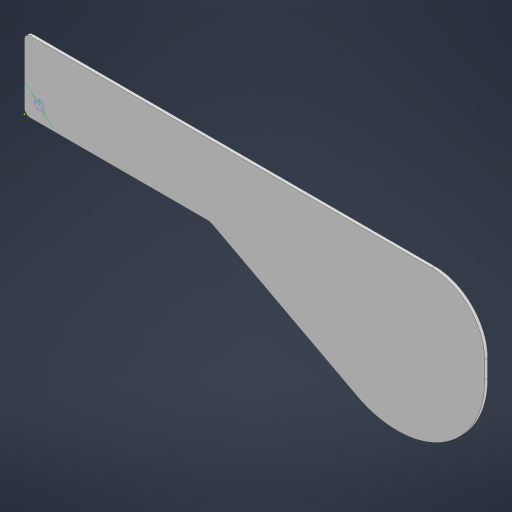
# Autodesk Inventor part: intake sled v5
Saved by Autodesk Inventor 2023.4 (Build 274418000, 418)
## iProperties
Created: 2023-12-16
Part Number: intake sled v5
Material: Generic
Document SubType Name: Modeling
Designer: Meer
Density: 1 g/cm^3
Appearance: Default
Author: Meer
Autodesk Inventor part; units mm, degrees
ref_plane "YZ Plane" through (0, 0, 0) normal (1, 0, 0) x (0, 1, 0)
ref_plane "XZ Plane" through (0, 0, 0) normal (0, 1, 0) x (-1, 0, 0)
ref_plane "XY Plane" through (0, 0, 0) normal (0, 0, 1) x (1, 0, 0)
sketch "Sketch1" plane through (0, 0, 0) normal (0, 0, 1) x (1, 0, 0)
  line L0 (0, 0) -> (247.65, 0)
  line L1 (247.65, 0) -> (247.65, 38.1)
  line L2 (247.65, 38.1) -> (0, 38.1)
  line L3 (0, 38.1) -> (0, 0)
  line L4 (286.1616, 0) -> (255.1962, 0)
  line L5 (255.1962, 0) -> (255.1962, 12.7)
  line L6 (255.1962, 12.7) -> (286.1616, 12.7)
  line L7 (286.1616, 12.7) -> (286.1616, 0)
  line L8 (247.65, 12.7) -> (200.66, 12.7)
  circle A0 centre (200.6294, 0) radius 47.0206
  line L9 (16.2468, 38.1) -> (16.2468, 12.7)
  line L10 (16.2468, 12.7) -> (155.3565, 12.7)
  line L11 (0, 12.7) -> (17.7951, 12.7)
  line L12 (179.5891, -42.0504) -> (75.8552, 12.7)
  point P0 (99.9175, 0)
  dimension "d0" = 247.65
  dimension "d1" = 38.1
  dimension "d2" = 12.7
  dimension "d3" = 30.9654
  dimension "d4" = 46.99
  dimension "d10" = 25.4
  constraints: 26 end point, 7 point on line, 5 perpendicular, 4 parallel, 3 point on circle, 2 horizontal, 1 centre point
  measures "d0" distance of L1.end L2.end
  measures "d1" distance of L0.end L1.end
  measures "d2" distance of L6.end L4.start
  measures "d3" distance of L5.end L6.end
  measures "d4" distance of L8.start L8.end
  measures "d10" distance of L9.start L9.end
extrude "Extrusion1" add sketch "Sketch1" along normal blind 1.5875 contours L3 L11 L10 L12 L0 | L12 L10 A0 L0 | L0 A0 L12 | L3 L2 L9 L11 | A0 L2 L0 | L0 A0 L12 | L10 L9 L2 A0 | A0 L8 L1 | L8 A0 L2 L1
fillet "Fillet1" radius 28.575 1 edges at (247.65, 38.1, 0.7937)
fillet "Fillet2" radius 3.175 1 edges at (0, 38.1, 0.7937)
fillet "Fillet4" radius 3.175 1 edges at (0, 0, 0.7937)
fillet "Fillet5" radius 5.08 1 edges at (99.9175, 0, 0.7937)
sketch "Sketch2" plane through (0, 0, 1.5875) normal (0, 0, 1) x (1, 0, 0)
  circle A0 centre (7.85, 8.4473) radius 2.54
  point P0 (0, 0)
  dimension "d13" = 5.08
  constraints: 1 centre point
  measures "d13" diameter of A0
body "Solid1"
